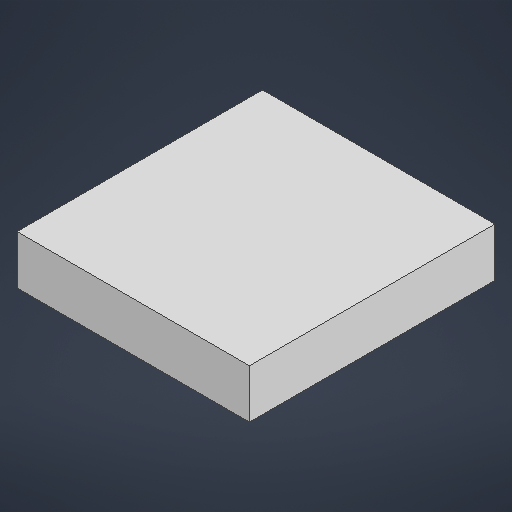
# Autodesk Inventor part: BLOK
Saved by Autodesk Inventor 2026 (Build 300175000, 175)
## iProperties
Created: 2025-04-11
Part Number: BLOK
Material: Generic
Document SubType Name: Modeling
Designer: janpa
Density: 1 g/cm^3
Appearance: Default
Author: janpa
Autodesk Inventor part; units mm, degrees
ref_plane "YZ Plane" through (0, 0, 0) normal (1, 0, 0) x (0, 1, 0)
ref_plane "XZ Plane" through (0, 0, 0) normal (0, 1, 0) x (-1, 0, 0)
ref_plane "XY Plane" through (0, 0, 0) normal (0, 0, 1) x (1, 0, 0)
sketch "Sketch1" plane through (0, 0, 0) normal (0, 1, 0) x (-1, 0, 0)
  line L0 (0, -0.2674) -> (4.7625, -0.2674)
  line L1 (4.7625, -0.2674) -> (4.7625, 4.7625)
  line L2 (4.7625, 4.7625) -> (0, 4.7625)
  line L3 (0, 4.7625) -> (0, -0.2674)
  point P0 (0, 0)
  constraints: 8 end point, 2 parallel, 1 horizontal, 1 perpendicular
extrude "Extrusion1" add sketch "Sketch1" along normal blind 1
body "Solid1"
